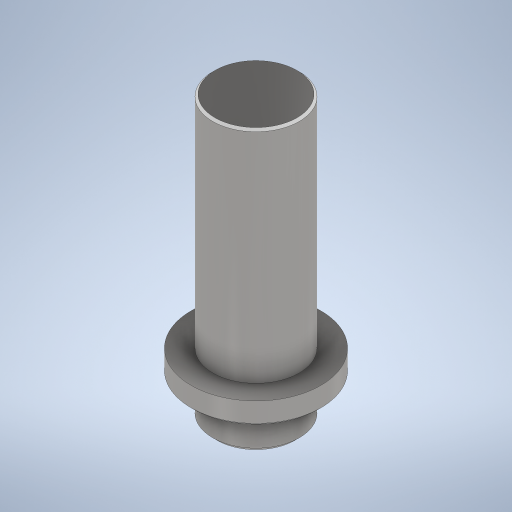
# Autodesk Inventor part: Khớp nối
Saved by Autodesk Inventor 2023 (Build 270158000, 158)
## iProperties
Created: 2023-10-05
Part Number: Khớp nối
Material: Generic
Document SubType Name: Modeling
Designer: huy20
Density: 1 g/cm^3
Appearance: Default
Author: huy20
Autodesk Inventor part; units mm, degrees
ref_plane "YZ Plane" through (0, 0, 0) normal (1, 0, 0) x (0, 1, 0)
ref_plane "XZ Plane" through (0, 0, 0) normal (0, 1, 0) x (-1, 0, 0)
ref_plane "XY Plane" through (0, 0, 0) normal (0, 0, 1) x (1, 0, 0)
sketch "Sketch1" plane through (0, 0, 0) normal (0, 0, 1) x (1, 0, 0)
  line L0 (0, 0) -> (0, 68.1171)
  line L1 (0, 34.0586) -> (2, 34.0586)
  line L2 (2, 34.0586) -> (2, 23.8615)
  line L3 (2, 23.8615) -> (3, 23.8615)
  line L4 (3, 23.8615) -> (3, 22.8615)
  line L5 (3, 22.8615) -> (2, 22.8615)
  line L6 (2, 22.8615) -> (2, 21.0586)
  line L7 (2, 21.0586) -> (0, 21.0586)
  point P0 (1, 21.0586)
  dimension "d0" = 13
  dimension "d1" = 1
  dimension "d2" = 6
  dimension "d3" = 2
  dimension "d4" = 4
  constraints: 16 end point, 5 perpendicular, 3 point on line, 2 midpoint, 1 horizontal, 1 vertical
  measures "d0" distance from line of point (1, 21.059) L1
  measures "d1" distance between parallel lines of L5 L3
  measures "d2" diameter of L4 L0
  measures "d3" distance of L6.end L7.end
  measures "d4" diameter of L6 L0
revolve "Revolution1" add sketch "Sketch1" angle 360 about axis through (0, 0, 0) along (0, 1, 0)
chamfer "Chamfer1" distance 0.2 angle 45 1 edges at (-2, 21.0586, 0)
chamfer "Chamfer2" distance 0.1 angle 45 1 edges at (-3, 22.8615, 0)
chamfer "Chamfer3" distance 0.1 angle 45 1 edges at (-2, 34.0586, 0)
body "Solid1"
